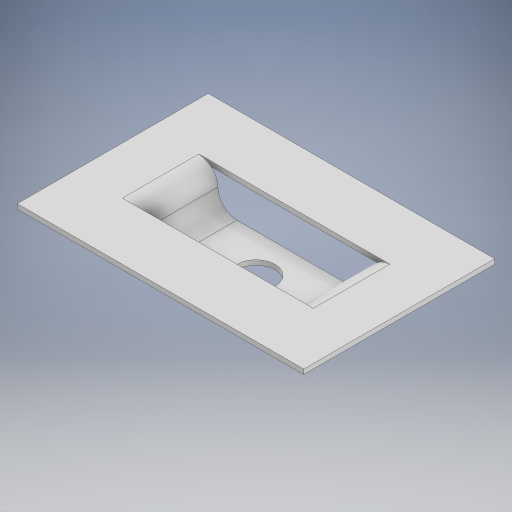
# Autodesk Inventor part: CE-4.1.3
Saved by Autodesk Inventor 2024 (Build 280153000, 153)
## iProperties
Created: 2024-02-08
Part Number: CE-4.1.3
Material: Generic
Document SubType Name: Sheet Metal
Designer: Alex
Density: 1 g/cm^3
Sheet Metal Rule: Default_mm
Appearance: Default
Author: Alex
Autodesk Inventor part; units mm, degrees
ref_plane "YZ Plane" through (0, 0, 0) normal (1, 0, 0) x (0, 1, 0)
ref_plane "XZ Plane" through (0, 0, 0) normal (0, 1, 0) x (-1, 0, 0)
sketch "Sketch1" plane through (0, 0, 0) normal (0, 1, 0) x (-1, 0, 0)
  line L0 (0, 0) -> (-30, 0)
  line L1 (-30, 0) -> (-30, -20)
  line L2 (-30, -20) -> (0, -20)
  line L3 (0, -20) -> (0, 0)
  dimension "d0" = 30
  dimension "d1" = 20
  measures "d0" distance of L2.end L1.end
  measures "d1" distance of L1.end L0.end
extrude "Plate1" add sketch "Sketch1" along normal blind 0.5
sketch "Sketch2" plane through (0, 0.5, 0) normal (0, 1, 0) x (1, 0, 0)
  line L0 (5, 14) -> (25, 14)
  line L1 (25, 14) -> (25, 6)
  line L2 (25, 6) -> (5, 6)
  line L3 (5, 6) -> (5, 14)
  line L4 (5, 14) -> (25, 6) construction
  line L5 (25, 14) -> (5, 6) construction
  line L6 (0, 0) -> (0, 20) projected
  line L7 (30, 0) -> (0, 0) projected
  point P0 (15, 10)
  dimension "d3" = 15
  dimension "d4" = 10
  dimension "d5" = 20
  dimension "Width" = 8
  constraints: 12 end point, 2 midpoint, 2 parallel, 1 horizontal, 1 perpendicular
  measures "d3" distance from line of point (15, 10) L6
  measures "d4" distance from line of L7 point (15, 10)
  measures "d5" distance of L0.start L0.end
  measures "Width" distance of L0.end L1.end
extrude "Extrusion1" cut sketch "Sketch2" against normal blind 0.5
ref_plane "Work Plane1" through (5, 0.5, -14) normal (0, 0, -1) x (-1, 0, 0)
sketch "Sketch3" plane through (5, 0.5, -14) normal (0, 0, -1) x (-1, 0, 0)
  line L0 (-20, 0) -> (0, 0) projected
  arc A0 (0, 0) -> (-2, -2) centre (0, -2) ccw
  arc A1 (-4, -4) -> (-2, -2) centre (-4, -2) ccw
  line L1 (-4, -4) -> (-16, -4)
  arc A2 (-18, -2) -> (-16, -4) centre (-16, -2) ccw
  arc A3 (-18, -2) -> (-20, 0) centre (-20, -2) ccw
  line L2 (0, 0) -> (-20, 0) projected
  arc A4 (-18.5, -2) -> (-20, -0.5) centre (-20, -2) ccw
  arc A5 (-18.5, -2) -> (-16, -4.5) centre (-16, -2) ccw
  line L3 (-16, -4.5) -> (-4, -4.5)
  arc A6 (-4, -4.5) -> (-1.5, -2) centre (-4, -2) ccw
  arc A7 (0, -0.5) -> (-1.5, -2) centre (0, -2) ccw
  line L4 (-20, -0.5) -> (-20, 0)
  line L5 (0, -0.5) -> (0, 0)
  point P0 (5, -0.5)
  dimension "d9" = 2
  dimension "d10" = 0.5
  constraints: 16 point on circle, 8 centre point, 8 end point, 6 tangent, 2 equal radius, 2 horizontal alignment, 2 vertical, 1 horizontal, 4 other
  measures "d9" radius of A0
  measures "d10" distance between parallel lines of L1 L3
extrude "Extrusion2" add sketch "Sketch3" against normal blind 8 contours A3 A2 L1 A1 A0 L5 A7 A6 L3 A5 A4 L4
sketch "Sketch4" plane through (9, -3.5, -14) normal (0, 1, 0) x (1, 0, 0)
  circle A0 centre (6, -4) radius 2
  point P0 (-9, -14)
  dimension "d13" = 4
  constraints: 1 centre point, 1 coincident
  measures "d13" diameter of A0
extrude "Extrusion3" cut sketch "Sketch4" against normal blind 0.5
equation "\"d7\" = Thickness"
equation "\"d10\" = Thickness"
equation "\"d11\" = Width"
equation "\"d14\" = Thickness"
equation "\"d2\" = Thickness"
equation "\"BendRadius\" = Thickness"
equation "\"BendReliefWidth\" = Thickness"
equation "\"BendReliefDepth\" = 0.5 * Thickness"
equation "\"CornerReliefSize\" = 4 * Thickness"
equation "\"MinimumRemnant\" = 2 * Thickness"
equation "\"TransitionRadius\" = BendRadius"
equation "\"JacobiRadiusSize\" = BendRadius"
equation "\"GapSize\" = Thickness"
equation "\"Thickness\" = 0.5"
body "Solid1"
